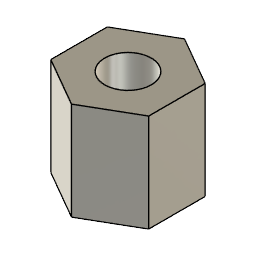
Acople ruedas (Autodesk Fusion 360 design; units mm, degrees)
Autodesk Fusion 360 part; units mm, degrees
sketch "Sketch1" plane through (0, 0, 0) normal (0, 0, 1) x (1, 0, 0)
  line L0 (-5.5, -3.1754) -> (0, -6.3509)
  line L1 (0, -6.3509) -> (5.5, -3.1754)
  line L2 (5.5, -3.1754) -> (5.5, 3.1754)
  line L3 (5.5, 3.1754) -> (0, 6.3509)
  line L4 (0, 6.3509) -> (-5.5, 3.1754)
  line L5 (-5.5, 3.1754) -> (-5.5, -3.1754)
  dimension "d1" = 5.5
  measures "d1" distance of origin L5
extrude "Extrude1" add sketch "Sketch1" along normal blind 5
sketch "Sketch2" plane through (0, 0, 5) normal (0, 0, 1) x (-1, 0, 0)
  line L0 (5.5, -3.1754) -> (5.5, 3.1754)
  line L1 (5.5, 3.1754) -> (0, 6.3509)
  line L2 (0, 6.3509) -> (-5.5, 3.1754)
  line L3 (-5.5, 3.1754) -> (-5.5, -3.1754)
  line L4 (-5.5, -3.1754) -> (0, -6.3509)
  line L5 (0, -6.3509) -> (5.5, -3.1754)
  circle A0 centre (0, 0) radius 2
  dimension "d4" = 4
  constraint coincident A0.centre origin
  measures "d4" diameter of A0
extrude "Extrude2" cut sketch "Sketch2" against normal blind 12 contours A0
extrude "Extrude3" add 1 faces at (-4.3333, 0, 5) along direction (0, 0, 1) blind 25
sketch "Sketch3" plane through (0, 0, 30) normal (0, 0, 1) x (-1, 0, 0)
  circle A0 centre (0, 0) radius 2
  line L0 (5.5, -3.1754) -> (5.5, 3.1754)
  line L1 (5.5, 3.1754) -> (0, 6.3509)
  line L2 (0, 6.3509) -> (-5.5, 3.1754)
  line L3 (-5.5, 3.1754) -> (-5.5, -3.1754)
  line L4 (-5.5, -3.1754) -> (0, -6.3509)
  line L5 (0, -6.3509) -> (5.5, -3.1754)
  line L6 (-5.8, -3.3486) -> (0, -6.6973)
  line L7 (0, -6.6973) -> (5.8, -3.3486)
  line L8 (5.8, -3.3486) -> (5.8, 3.3486)
  line L9 (5.8, 3.3486) -> (0, 6.6973)
  line L10 (0, 6.6973) -> (-5.8, 3.3486)
  line L11 (-5.8, 3.3486) -> (-5.8, -3.3486)
  dimension "d9" = 5.8
  constraint coincident A0.centre origin
  measures "d9" distance of A0.centre L11
extrude "Extrude4" add sketch "Sketch3" against normal blind 16 contours L6 L7 L8 L9 L10 L11
sketch "Sketch4" plane through (0, 0, 30) normal (0, 0, 1) x (-1, 0, 0)
  line L0 (-5.8, 3.3486) -> (-5.8, -3.3486)
  line L1 (-5.8, -3.3486) -> (0, -6.6973)
  line L2 (0, -6.6973) -> (5.8, -3.3486)
  line L3 (5.8, -3.3486) -> (5.8, 3.3486)
  line L4 (5.8, 3.3486) -> (0, 6.6973)
  line L5 (0, 6.6973) -> (-5.8, 3.3486)
  circle A0 centre (0, 0) radius 2
  circle A1 centre (0, 0) radius 2.65
  dimension "d12" = 5.3
  constraint coincident A0.centre A1.centre
  measures "d12" diameter of A1
extrude "Extrude5" cut sketch "Sketch4" against normal blind 35 contours A1
extrude "Extrude6" cut 1 faces at (-2.275, -3.9404, 0) along direction (0, 0, 1) blind 2
extrude "Extrude7" cut 1 faces at (2.375, -4.1136, 30) along direction (0, 0, -1) blind 33 from surface at 12
sketch "Sketch5" plane through (0, 0, 30) normal (0, 0, 1) x (-1, 0, 0)
  circle A0 centre (0, 0) radius 2.65
  line L0 (-5.8, 3.3486) -> (-5.8, -3.3486)
  line L1 (-5.8, -3.3486) -> (0, -6.6973)
  line L2 (0, -6.6973) -> (5.8, -3.3486)
  line L3 (5.8, -3.3486) -> (5.8, 3.3486)
  line L4 (5.8, 3.3486) -> (0, 6.6973)
  line L5 (0, 6.6973) -> (-5.8, 3.3486)
  line L6 (-6.1, -3.5218) -> (0, -7.0437)
  line L7 (0, -7.0437) -> (6.1, -3.5218)
  line L8 (6.1, -3.5218) -> (6.1, 3.5218)
  line L9 (6.1, 3.5218) -> (0, 7.0437)
  line L10 (0, 7.0437) -> (-6.1, 3.5218)
  line L11 (-6.1, 3.5218) -> (-6.1, -3.5218)
  dimension "d20" = 6.1
  constraint coincident A0.centre origin
  measures "d20" distance of A0.centre L11
extrude "Extrude8" add sketch "Sketch5" against normal blind 12 contours L6 L7 L8 L9 L10 L11
sketch "Sketch6" plane through (0, 0, 30) normal (0, 0, 1) x (-1, 0, 0)
  line L0 (-6.1, 3.5218) -> (-6.1, -3.5218)
  line L1 (-6.1, -3.5218) -> (0, -7.0437)
  line L2 (0, -7.0437) -> (6.1, -3.5218)
  line L3 (6.1, -3.5218) -> (6.1, 3.5218)
  line L4 (6.1, 3.5218) -> (0, 7.0437)
  line L5 (0, 7.0437) -> (-6.1, 3.5218)
  circle A0 centre (0, 0) radius 2.65
  line L6 (-6, -3.4641) -> (0, -6.9282)
  line L7 (0, -6.9282) -> (6, -3.4641)
  line L8 (6, -3.4641) -> (6, 3.4641)
  line L9 (6, 3.4641) -> (0, 6.9282)
  line L10 (0, 6.9282) -> (-6, 3.4641)
  line L11 (-6, 3.4641) -> (-6, -3.4641)
  circle A1 centre (0, 0) radius 2.85
  dimension "d23" = 6
  dimension "d24" = 5.7
  constraint coincident A0.centre A1.centre
  measures "d23" distance of A0.centre L11
  measures "d24" diameter of A1
extrude "Extrude9" cut sketch "Sketch6" against normal blind 13
